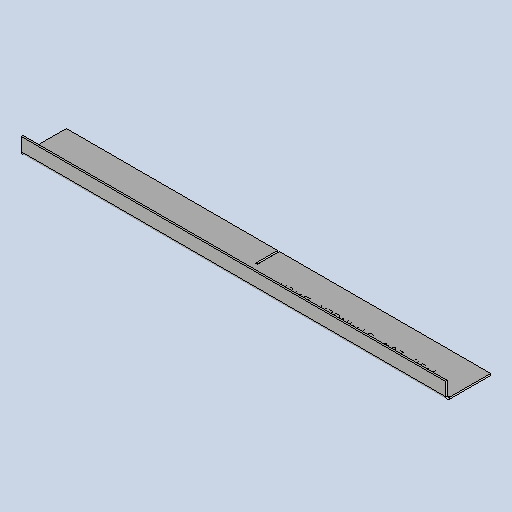
# Autodesk Inventor part: MSC 204 STRINGER BACK ^
Saved by Autodesk Inventor 2025.1 (Build 291241020, 241B)
## iProperties
Created: 2024-04-28
Part Number: MSC 204 STRINGER BACK ^
Material: Stainless Steel
Document SubType Name: Sheet Metal
Designer: admin
Stock Number: МОО 204 стрингер спина ^
Density: 8 g/cm^3
Flat Pattern Width: 49 cm
Flat Pattern Length: 6.8202 cm
Flat Pattern Area: 334.19 cm^2
Sheet Metal Rule: AISI304 2mm Die16
Sheet Metal Width: 490.000 mm
Sheet Metal Length: 68.202 mm
Sheet Metal Area: 33418.975 mm^2
Appearance: Default
Mass: 535.409 g
Surface Area: 692.516 cm^2
Volume: 66.9261 cm^3
Author: admin
Autodesk Inventor part; units mm, degrees
ref_plane "YZ Plane" through (0, 0, 0) normal (1, 0, 0) x (0, 1, 0)
ref_plane "XZ Plane" through (0, 0, 0) normal (0, 1, 0) x (-1, 0, 0)
ref_plane "XY Plane" through (0, 0, 0) normal (0, 0, 1) x (1, 0, 0)
sketch "Sketch1" plane through (0, 0, 0) normal (0, 0, 1) x (1, 0, 0)
  line L0 (-490, 52) -> (490, 52)
  line L1 (490, 52) -> (490, 0)
  line L2 (490, 0) -> (-490, 0)
  line L3 (-490, 0) -> (-490, 52)
  point P0 (0, 0)
  point P1 (0, 0)
  dimension "d0" = 980
  dimension "d1" = 52
  measures "d0" distance of L1.end L2.end
  measures "d1" distance of L0.end L1.end
extrude "Plate1" add sketch "Sketch1" along normal blind 2
sketch "Sketch2" plane through (490, 2, 0) normal (0, -1, 0) x (1, 0, 0)
  line L0 (-980, 0) -> (0, 0)
  line L1 (0, 0) -> (0, 20)
  line L2 (0, 20) -> (-980, 20)
  line L3 (-980, 20) -> (-980, 0)
  constraints: 6 end point, 1 horizontal, 1 perpendicular, 1 vertical
edge flange "Flange1" height 20 angle 90 thickness 2 bend radius 2.75 thickness toward (0, -1, 0) relief round relief width 2 relief depth 1 edges at (0, 0, 2) wall of the first edge with corners at (-490, 2, 0) (490, 2, 0) (490, 2, 20) (-490, 2, 20)
bend "Bend1"
corner "Corner1"
sketch "Sketch11" plane through (0, 0, 0) normal (0, 0, 1) x (1, 0, 0)
  line L0 (-490, 52) -> (490, 52) projected
  circle A0 centre (0, 52) radius 30
  line L1 (-490, 0) -> (490, 0) projected
  line L2 (246.05, 0) -> (243.95, 0)
  line L3 (243.95, 0) -> (243.95, 27)
  line L4 (243.95, 27) -> (246.05, 27)
  line L5 (246.05, 27) -> (246.05, 0)
  line L6 (-243.95, 0) -> (-246.05, 0)
  line L7 (-246.05, 0) -> (-246.05, 27) construction
  line L8 (-246.05, 27) -> (-243.95, 27) construction
  line L9 (-243.95, 27) -> (-243.95, 0) construction
  line L10 (0, 52) -> (0, 0)
  line L11 (246.05, 27) -> (246.05, 52)
  line L12 (243.95, 27) -> (243.95, 52)
  line L13 (-243.95, 27) -> (-243.95, 52) construction
  line L14 (-246.05, 27) -> (-246.05, 52) construction
  line L15 (-490, 0) -> (-490, 52)
  circle A1 centre (490, 52) radius 30
  line L16 (490, 52) -> (490, 0)
  point P0 (30, 52)
  point P1 (-30, 52)
  point P2 (-245, 27)
  point P3 (245, 27)
  point P4 (490, 22)
  point P5 (460, 52)
  point P6 (0, 22)
  dimension "d44" = 60
  dimension "d47" = 2.1
  dimension "d49" = 490
  dimension "d50" = 27
  constraints: 30 end point, 8 perpendicular, 7 point on line, 4 parallel, 3 midpoint, 2 centre point, 2 horizontal, 1 coincident, 1 collinear, 1 equal radius, 1 vertical, 1 other
  measures "d44" diameter of A0
  measures "d47" distance of L3.end L4.end
  measures "d49" distance of point (-245, 27) point (245, 27)
  measures "d50" distance between parallel lines of L1 L4
extrude "Extrusion4" cut sketch "Sketch11" along normal through all both and the other way through all contours L10 A0 L0 | A0 L10 L1 L15 L0 | L0 L11 L4 L12 picked at (-19.7493, 49.7748)
sketch "Sketch9" plane through (0, 0, 2) normal (0, 0, 1) x (1, 0, 0)
  line L0 (456.3279, 23.6801) -> (456.3279, 11.6801) construction
  line L1 (456.3279, 11.6801) -> (256.3279, 11.6801) construction
  line L2 (256.3279, 11.6801) -> (256.3279, 23.6801) construction
  line L3 (256.3279, 23.6801) -> (456.3279, 23.6801) construction
  line L4 (-490, 52) -> (490, 52) projected
  point P0 (0, 0)
  point P1 (1, 52)
  dimension "d38" = 200
  dimension "d39" = 12
  constraints: 1 horizontal, 2 other
  measures "d38" distance of L0.end L1.end
  measures "d39" distance of L1.end L2.end
mark "Mark3"
equation "\"d1\" = СПИНА_Стрингер_1_высота"
equation "\"d2\" = Thickness"
equation "\"d3\" = BendReliefWidth"
equation "\"d4\" = BendReliefDepth"
equation "\"d5\" = MinimumRemnant"
equation "\"d6\" = TransitionRadius"
equation "\"d9\" = BendRadius"
equation "\"d10\" = CornerReliefSize"
equation "\"d11\" = GapSize"
equation "\"d12\" = JacobiRadiusSize"
equation "\"BendReliefWidth\" = Thickness"
equation "\"BendReliefDepth\" = 0.5 * Thickness"
equation "\"CornerReliefSize\" = 4 * Thickness"
equation "\"MinimumRemnant\" = 2 * Thickness"
equation "\"TransitionRadius\" = BendRadius"
equation "\"JacobiRadiusSize\" = BendRadius"
equation "\"GapSize\" = Thickness"
equation "\"СПИНА_Стрингер_1_высота\" = 52"
equation "\"Thickness\" = 2"
equation "\"BendRadius\" = 2.75"
body "Solid1"
